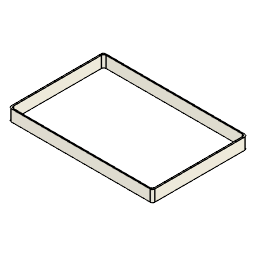
center1 (Autodesk Fusion 360 design; units mm, degrees)
part number: 2025-09-30-18-53-28-818
Autodesk Fusion 360 part; units mm, degrees
sketch "Sketch1" plane through (0, 0, 0) normal (0, 0, 1) x (1, 0, 0)
  line L0 (5.4842, 0) -> (306.4842, 0)
  line L1 (311.4842, 5) -> (311.4842, 200)
  line L2 (306.4842, 205) -> (5.4842, 205)
  line L3 (0.4842, 200) -> (0.4842, 5)
  line L4 (8.4842, 2.5) -> (303.4842, 2.5)
  line L5 (308.4842, 7.5) -> (308.4842, 197.5)
  line L6 (303.4842, 202.5) -> (8.4842, 202.5)
  line L7 (3.4842, 197.5) -> (3.4842, 7.5)
  arc A0 (8.4842, 202.5) -> (3.4842, 197.5) centre (8.4842, 197.5) ccw
  arc A1 (5.4842, 205) -> (0.4842, 200) centre (5.4842, 200) ccw
  arc A2 (308.4842, 197.5) -> (303.4842, 202.5) centre (303.4842, 197.5) ccw
  arc A3 (311.4842, 200) -> (306.4842, 205) centre (306.4842, 200) ccw
  arc A4 (3.4842, 7.5) -> (8.4842, 2.5) centre (8.4842, 7.5) ccw
  arc A5 (0.4842, 5) -> (5.4842, 0) centre (5.4842, 5) ccw
  arc A6 (303.4842, 2.5) -> (308.4842, 7.5) centre (303.4842, 7.5) ccw
  arc A7 (306.4842, 0) -> (311.4842, 5) centre (306.4842, 5) ccw
  point P0 (0.4842, 0)
  point P1 (311.4842, 0)
  point P2 (3.4842, 2.5)
  point P3 (308.4842, 2.5)
  dimension "d1" = 311
  dimension "d2" = 205
  dimension "d3" = 305
  dimension "d4" = 200
  dimension "d5" = 2.5
  dimension "d6" = 2.5
  dimension "d7" = 3
  dimension "d8" = 3
  dimension "d9" = 5
  dimension "d10" = 5
  dimension "d11" = 5
  dimension "d12" = 5
  dimension "d13" = 5
  dimension "d14" = 5
  dimension "d15" = 5
  dimension "d16" = 5
  constraint horizontal L0
  constraint vertical L1
  constraint horizontal L2
  constraint vertical L3
  constraint horizontal L4
  constraint vertical L5
  constraint horizontal L6
  constraint vertical L7
  constraint tangent L6 A0
  constraint tangent L7 A0
  constraint tangent L2 A1
  constraint tangent L3 A1
  constraint tangent L5 A2
  constraint tangent L6 A2
  constraint tangent L1 A3
  constraint tangent L2 A3
  constraint coincident P2 L4
  constraint coincident P2 L7
  constraint tangent L4 A4
  constraint tangent L7 A4
  constraint coincident P0 L0
  constraint coincident P0 L3
  constraint tangent L0 A5
  constraint tangent L3 A5
  constraint coincident P3 L4
  constraint coincident P3 L5
  constraint tangent L4 A6
  constraint tangent L5 A6
  constraint coincident P1 L0
  constraint coincident P1 L1
  constraint tangent L0 A7
  constraint tangent L1 A7
  measures "d1" distance of P0 P1
  measures "d2" distance of L0 L2
  measures "d3" distance of P2 P3
  measures "d4" distance of L4 L6
  measures "d5" distance of L0 L4
  measures "d6" distance of L2 L6
  measures "d7" distance of L3 L7
  measures "d8" distance of L1 L5
  measures "d9" radius of A0
  measures "d10" radius of A1
  measures "d11" radius of A2
  measures "d12" radius of A3
  measures "d13" radius of A4
  measures "d14" radius of A5
  measures "d15" radius of A6
  measures "d16" radius of A7
extrude "Extrude1" add sketch "Sketch1" along normal blind 25
